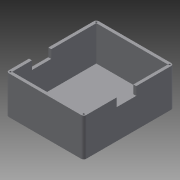
# Autodesk Inventor part: MotorDriverModel
Saved by Autodesk Inventor 2015 (Build 190159000, 159)
## iProperties
Created: 2015-09-03
Part Number: MotorDriverModel
Material: Generic
Document SubType Name: Modeling
Designer: Lauszus
Density: 1 g/cm^3
Appearance: Default
Author: Lauszus
Autodesk Inventor part; units mm, degrees
ref_plane "YZ Plane" through (0, 0, 0) normal (1, 0, 0) x (0, 1, 0)
ref_plane "XZ Plane" through (0, 0, 0) normal (0, 1, 0) x (-1, 0, 0)
ref_plane "XY Plane" through (0, 0, 0) normal (0, 0, 1) x (1, 0, 0)
sketch "Sketch2" plane through (0, 0, 0) normal (0, 1, 0) x (-1, 0, 0)
  line L0 (35.0336, 55.0564) -> (-56.9664, 55.0564)
  line L1 (-56.9664, 55.0564) -> (-56.9664, -51.9436)
  line L2 (-56.9664, -51.9436) -> (35.0336, -51.9436)
  line L3 (35.0336, -51.9436) -> (35.0336, 55.0564)
  point P0 (0, 0)
  dimension "d28" = 107
  dimension "d29" = 92
  constraints: 8 end point, 2 parallel, 1 horizontal, 1 perpendicular
  measures "d28" distance of L2.end L0.start
  measures "d29" distance of L1.end L2.end
extrude "Extrusion2" add sketch "Sketch2" along normal blind 45
shell "Shell2" thickness 3.5 removed faces 1 at (-4.367, 45, -16.277)
fillet "Fillet1" radius 3 4 edges at (56.9664, 22.5, 55.0564) (-35.0336, 22.5, 55.0564) (56.9664, 22.5, -51.9436) (-35.0336, 22.5, -51.9436)
sketch "Sketch3" plane through (0, 45, 0) normal (0, 1, 0) x (1, 0, 0)
  circle A0 centre (54.4664, -52.5564) radius 1
  line L0 (-32.0336, -55.0564) -> (53.9664, -55.0564) projected
  line L1 (56.9664, -52.0564) -> (56.9664, 48.9436) projected
  line L2 (10.9664, -40.0013) -> (10.9664, -71.8309)
  line L3 (-21.6043, -1.5564) -> (-51.5358, -1.5564)
  circle A1 centre (-32.5336, -52.5564) radius 1
  circle A2 centre (54.4664, 49.4436) radius 1
  circle A3 centre (-32.5336, 49.4436) radius 1
  point P0 (0, 0)
  dimension "d34" = 2
  dimension "d35" = 2.5
  dimension "d36" = 2.5
  dimension "d37" = 46
  dimension "d38" = 53.5
  constraints: 4 centre point, 4 end point, 3 symmetric about line, 1 horizontal, 1 vertical, 3 other
  measures "d34" diameter of A0
  measures "d35" distance from line of L0 A0.centre
  measures "d36" distance from line of L1 A0.centre
  measures "d37" distance between parallel lines of L1 L2
  measures "d38" distance between parallel lines of L0 L3
extrude "Extrusion3" cut sketch "Sketch3" against normal blind 7
sketch "Sketch9" plane through (56.9664, 0, 52.0564) normal (1, 0, 0) x (0, 0, -1)
  line L0 (59.45, 45) -> (36.05, 45)
  line L1 (36.05, 45) -> (36.05, 35)
  line L2 (36.05, 35) -> (59.45, 35)
  line L3 (59.45, 35) -> (59.45, 45)
  line L4 (-3, 45) -> (-3, 0) projected
  line L5 (104, 0) -> (104, 45) projected
  line L6 (0, 45) -> (101, 45) projected
  point P0 (52.0564, 0)
  point P1 (-3, 2)
  point P2 (107, 2)
  dimension "d102" = 10
  dimension "d103" = 39.05
  dimension "d104" = 44.55
  dimension "d105" = 0
  constraints: 8 end point, 2 parallel, 1 horizontal, 1 perpendicular, 1 other
  measures "d102" distance of L2.end L0.start
  measures "d103" distance between parallel lines of L4 L1
  measures "d105" distance between parallel lines of L0 L6
extrude "Extrusion5" cut sketch "Sketch9" against normal blind 8
sketch "Sketch10" plane through (-35.0336, 0, -48.9436) normal (-1, 0, 0) x (0, 0, 1)
  line L0 (54.05, 35) -> (76.95, 35)
  line L1 (76.95, 35) -> (76.95, 45)
  line L2 (76.95, 45) -> (54.05, 45)
  line L3 (54.05, 45) -> (54.05, 35)
  line L4 (104, 0) -> (104, 45) projected
  line L5 (0, 45) -> (101, 45) projected
  line L6 (-3, 45) -> (-3, 0) projected
  point P0 (48.9436, 0)
  point P1 (107, 2)
  point P2 (-3, 2)
  dimension "d108" = 27.05
  dimension "d109" = 0
  dimension "d110" = 57.05
  dimension "d111" = 10
  constraints: 8 end point, 2 parallel, 1 horizontal, 1 perpendicular, 1 other
  measures "d109" distance between parallel lines of L2 L5
  measures "d110" distance between parallel lines of L3 L6
  measures "d111" distance of L2.end L0.start
extrude "Extrusion6" cut sketch "Sketch10" against normal blind 8
body "Solid2"
